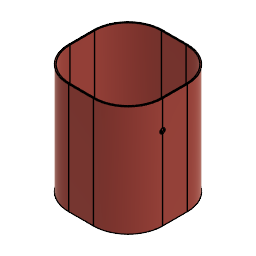
OuterShell_v5 (Autodesk Fusion 360 design; units mm, degrees)
Autodesk Fusion 360 part; units mm, degrees
note: some values were not read from the file. Set by a fixed rule: which sketch regions a step uses; which face or edge a step refers to.
sketch "Sketch1" plane through (0, 0, 0) normal (0, 0, 1) x (1, 0, 0)
  line L0 (55, -55) -> (-55, -55)
  line L1 (-55, -55) -> (-55, 55)
  line L2 (-55, 55) -> (55, 55)
  line L3 (55, 55) -> (55, -55)
  line L4 (55, -55) -> (-55, 55) construction
  line L5 (-55, -55) -> (55, 55) construction
  dimension "d1" = 110
  dimension "d2" = 110
  constraint horizontal L0
  constraint perpendicular L0 L1
  constraint parallel L0 L2
  constraint parallel L1 L3
  constraint coincident L4 origin
  constraint coincident L5 origin
  measures "d1" distance of L1.end L2.end
  measures "d2" distance of L0.end L1.end
extrude "Extrude1" add sketch "Sketch1" along normal blind 134
fillet "Fillet1" radius 42 4 edges at (55, -55, 67) (55, 55, 67) (-55, 55, 67) (-55, -55, 67)
move_face "OffsetFaces1" offset 2 4 faces at (-4.3333, 55, 44.6667) (55, 4.3333, 44.6667) (4.3333, -55, 44.6667) (-55, -4.3333, 44.6667)
shell "Shell1" thickness 1.5 removed faces 1 at (-19, 5, 134)
sketch "Sketch3" plane through (57, 0, 0) normal (1, 0, 0) x (0, 1, 0)
  line L0 (-15, 134) -> (-15, 0)
  line L1 (-15, 0) -> (15, 0)
  line L2 (15, 0) -> (15, 134)
  line L3 (15, 134) -> (-15, 134)
  circle A0 centre (-15, 100) radius 3
  dimension "d12" = 6
  constraint coincident L0 A0.centre
  measures "d12" diameter of A0
extrude "Extrude3" cut sketch "Sketch3" against normal blind 10 contours L0 A0 | L0 A0
sketch "Sketch4" plane through (-57, 0, 0) normal (-1, 0, 0) x (0, -1, 0)
  line L0 (15, 0) -> (15, 134)
  line L1 (15, 134) -> (-15, 134)
  line L2 (-15, 134) -> (-15, 0)
  line L3 (-15, 0) -> (15, 0)
  circle A0 centre (18.3132, 22.5159) radius 10
  dimension "d15" = 20
  measures "d15" diameter of A0
extrude "Extrude4" cut sketch "Sketch4" against normal blind 5 contours L0 A0 | L0 A0
